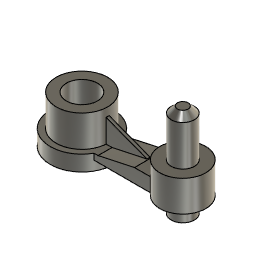
Tarea09_Ej3_jaalobuela (Autodesk Fusion 360 design; units mm, degrees)
Autodesk Fusion 360 part; units mm, degrees
sketch "Sketch1" plane through (0, 0, 0) normal (0, 0, 1) x (1, 0, 0)
  circle A0 centre (-15, 20) radius 8.295
  circle A1 centre (-15, 20) radius 10.195
  line L0 (-15, 20) -> (20.52, 20)
  circle A2 centre (20.52, 20) radius 3.745
  dimension "d1" = 16.59
  dimension "d2" = 20.39
  dimension "d3" = 35.52
  dimension "d4" = 7.49
  constraint concentric A0 A1
  constraint coincident A0.centre A1.centre
  constraint horizontal L0
  constraint coincident L0.end A2.centre
  measures "d1" diameter of A0
  measures "d2" diameter of A1
  measures "d3" distance of A0.centre L0.end
  measures "d4" diameter of A2
extrude "Extrude1" add sketch "Sketch1" along normal blind 5 contours A0 | A1 makes body 1
sketch "Sketch2" plane through (0, 0, 5) normal (0, 0, 1) x (-1, 0, 0)
  circle A0 centre (15, -20) radius 10.195
  circle A1 centre (15, -20) radius 8.295
  dimension "d8" = 16.59
  constraint concentric A0 A1
  measures "d8" diameter of A1
extrude "Extrude2" add sketch "Sketch1" along normal blind 5 separate body contours A2 makes body 2
sketch "Sketch3" plane through (0, 0, 0) normal (0, 0, 1) x (1, 0, 0)
sketch "Sketch4" plane through (0, 0, 0) normal (0, 0, 1) x (1, 0, 0)
sketch "Sketch5" plane through (0, 0, 5) normal (0, 0, 1) x (1, 0, 0)
  circle A0 centre (-15, 20) radius 5
  dimension "d13" = 10
  measures "d13" diameter of A0
sketch "Sketch6" plane through (0, 0, 0) normal (0, 1, 0) x (1, 0, 0)
  circle A0 through (28.49, -40, 0) (25.8725, -40, -1.5112) (25.8725, -40, 1.5112)
  circle A1 through (30.49, -38.0003, 0) (24.8725, -38.0003, -3.2433) (24.8725, -38.0003, 3.2433)
  line L0 (26.745, -40) -> (26.745, -38.0003)
loft "Loft1" add profiles "Sketch6", "Sketch6" section 1 contours A0 in plane through (0, 0, 40) normal (0, 0, -1) section 2 contours A1 in plane through (0, 0, 38.0003) normal (0, 0, -1) separate body makes body 3
extrude "Extrude3" add sketch "Sketch6" along normal blind 13 contours A1 in plane through (0, 0, 38.0003) normal (0, 0, -1) bodies 3
sketch "Sketch7" plane through (0, 0, 0) normal (0, 0, 1) x (1, 0, 0)
  circle A0 centre (48, 1) radius 7.385
  dimension "d21" = 14.77
  measures "d21" diameter of A0
extrude "Extrude4" add sketch "Sketch7" along normal blind 10 separate body makes body 4
move_body "Move1" bodies 4 to x (1, 0, 0) y (0, 1, 0) z (0, 0, 1) at (-21.255, -1, 15.0003)
move_body "Move2" bodies 2 to x (1, 0, 0) y (0, 1, 0) z (0, 0, 1) at (6.225, -20, 10.0003)
move_body "Move3" bodies 2 3 4 to x (1, 0, 0) y (0, 1, 0) z (0, 0, 1) at (-6.225, 20, -10.0003)
sketch "Sketch8" plane through (0, 0, 0) normal (0, 0, 1) x (1, 0, 0)
  line L0 (4, 38) -> (14.58, 38)
  line L1 (14.58, 38) -> (14.58, 28)
  line L2 (14.58, 28) -> (4, 28)
  line L3 (4, 28) -> (4, 38)
  line L4 (15.0651, 15) -> (9.92, 15)
  line L5 (9.92, 15) -> (9.92, 25)
  line L6 (9.92, 25) -> (15.0651, 25)
  circle A0 centre (20.5, 20) radius 7.385
  dimension "d24" = 10.58
  dimension "d25" = 10
  dimension "d28" = 10
  dimension "d31" = 14.77
  dimension "d46" = 10.58
  constraint horizontal L0
  constraint vertical L1
  constraint horizontal L2
  constraint vertical L3
  constraint perpendicular L4 L5
  constraint perpendicular L5 L6
  constraint coincident A0 L6.end
  constraint coincident A0 L4.start
  measures "d24" distance of L0.start L0.end
  measures "d25" distance of L0.start L2.end
  measures "d28" distance of L4.end L5.end
  measures "d31" diameter of A0
  measures "d46" distance of L5 A0.centre
sketch "Sketch9" plane through (0, 0, 0) normal (0, 1, 0) x (1, 0, 0)
  line L0 (13, -5) -> (12.3205, -5)
  line L1 (12.3205, -5) -> (12.3205, -5.53)
  dimension "d30" = 0.53
  constraint horizontal L0
  constraint perpendicular L0 L1
  measures "d30" distance of L0.end L1.end
extrude "Extrude5" add sketch "Sketch8" along normal blind 4.47 separate body contours L4 L5 L6 A0 makes body 5
move_body "Move4" bodies 5 to x (1, 0, 0) y (0, 1, 0) z (0, 0, 1) at (0, 0, 5.53)
sketch "Sketch10" plane through (0, 0, 5) normal (0, 0, 1) x (-1, 0, 0)
  circle A0 centre (15, -20) radius 10.195
  circle A1 centre (15, -20) radius 5
  dimension "d37" = 10
  constraint concentric A0 A1
  measures "d37" diameter of A1
extrude "Extrude6" add sketch "Sketch10" along normal blind 10 contours A1 bodies 1
sketch "Sketch11" plane through (0, 0, 0) normal (0, 1, 0) x (1, 0, 0)
  line L0 (9.92, -5.53) -> (-1.83, -5.53)
  line L1 (9.92, -5.53) -> (9.92, -10)
  line L2 (-1.83, -5.53) -> (-1.83, -7.47)
  line L3 (-1.83, -7.47) -> (9.92, -10)
  dimension "d40" = 11.75
  dimension "d43" = 1.94
  constraint horizontal L0
  constraint perpendicular L0 L1
  constraint perpendicular L0 L2
  measures "d40" distance of L0.start L0.end
  measures "d43" distance of L0.end L2.end
extrude "Extrude7" add sketch "Sketch11" along normal blind 10 separate body makes body 6
move_body "Move5" bodies 6 to x (1, 0, 0) y (0, 1, 0) z (0, 0, 1) at (0, 15, 0)
sketch "Sketch12" plane through (0, 0, 5) normal (0, 0, 1) x (-1, 0, 0)
  circle A0 centre (15, -20) radius 5
  circle A1 centre (15, -20) radius 10.195
  line L0 (15, -20) -> (15, -25)
  line L1 (15, -20) -> (15, -15)
  line L2 (6.1153, -15) -> (1.83, -15)
  line L3 (15, -20) -> (-20.52, -20)
  line L4 (6.1153, -25) -> (1.83, -25)
  arc A2 (6.1153, -15) -> (6.1153, -25) centre (15, -20) ccw
  line L5 (1.83, -15) -> (1.83, -25)
  dimension "d47" = 5
  dimension "d48" = 5
  constraint concentric A0 A2
  constraint coincident A0.centre A1.centre
  constraint vertical L0
  constraint parallel L0 L1
  constraint tangent A0 L2
  constraint perpendicular L1 L2
  constraint symmetric L2.end L3 L4.end
  constraint coincident A1 L4.start
  constraint perpendicular L4 L5
  measures "d47" distance of A0.centre L0.end
  measures "d48" distance of A0.centre L1.end
extrude "Extrude8" add sketch "Sketch12" along normal blind 1.94 separate body contours A1 L2 L3 A2 L5 | A1 L3 L4 A2 L5 makes body 7
move_body "Move6" bodies 7 to x (1, 0, 0) y (0, 1, 0) z (0, 0, 1) at (0, 0, 0.53)
move_body "Move7" bodies 1 to x (1, 0, 0) y (0, 1, 0) z (0, 0, 1) at (0, 0, 2.47)
extrude "Extrude9" add sketch "Sketch1" along normal blind 10 separate body contours A0 makes body 8
move_body "Move8" bodies 8 to x (1, 0, 0) y (0, 1, 0) z (0, 0, 1) at (0, 0, 7.47)
combine "Combine1" operation cut target body 8 tool bodies 1
extrude "Extrude10" add sketch "Sketch1" along normal blind 5 separate body contours A0 | A1 makes body 9
move_body "Move9" bodies 9 to x (1, 0, 0) y (0, 1, 0) z (0, 0, 1) at (0, 0, 2.47)
sketch "Sketch13" plane through (0, 0, 0) normal (0, 1, 0) x (1, 0, 0)
  line L0 (20.52, 0) -> (20.52, 1.5)
  line L1 (20.52, 1.5) -> (9.46, 1.5)
  line L2 (9.46, 1.5) -> (9.46, -12.5848)
  line L3 (-25.195, -2.47) -> (-25.195, -14.93)
  line L4 (-25.195, -14.93) -> (-6.7, -14.93)
  line L5 (-6.7, -14.93) -> (-6.7, -7.47)
  line L6 (-6.7, -7.47) -> (-1.83, -7.47)
  line L7 (-1.83, -7.47) -> (9.46, -9.901)
  line L8 (-6.7, -14.93) -> (9.46, -9.901)
  dimension "d55" = 11.06
  dimension "d56" = 12.46
  dimension "d57" = 7.46
  constraint vertical L0
  constraint perpendicular L0 L1
  constraint perpendicular L1 L2
  constraint vertical L3
  constraint perpendicular L3 L4
  constraint perpendicular L4 L5
  constraint perpendicular L5 L6
  constraint coincident L2 L7.end
  measures "d55" distance of L0.end L1.end
  measures "d56" distance of L3.start L3.end
  measures "d57" distance of L4.end L5.end
extrude "Extrude11" add sketch "Sketch13" along normal blind 1 separate body makes body 10
move_body "Move10" bodies 10 to x (1, 0, 0) y (0, 1, 0) z (0, 0, 1) at (0, 19.5, 0)
copy_body "CopyPasteBodies1" bodies 8 10 3 9 4 2 5 7 6 makes body 11 makes body 12 makes body 13 makes body 14 makes body 15 makes body 16 makes body 17 makes body 18 makes body 19
move_body "Move11" bodies 11 12 13 14 15 16 17 18 19 to x (1, 0, 0) y (0, 1, 0) z (0, 0, 1) at (74, 0, 0)
move_body "Move12" bodies 11 14 to x (1, 0, 0) y (0, 1, 0) z (0, 0, 1) at (2.98, 0, 0)
move_body "Move13" bodies 3 to x (1, 0, 0) y (0, 1, 0) z (0, 0, 1) at (0, 0, 9)
move_body "Move14" bodies 3 to x (1, 0, 0) y (0, 1, 0) z (0, 0, 1) at (0, 0, -9)
combine "Combine2" operation add target body 19 tool bodies 11 18 14 17 12
move_body "Move15" bodies 4 2 3 to x (1, 0, 0) y (0, 1, 0) z (0, 0, 1) at (123, 0, 0)
copy_body "CopyPasteBodies2" bodies 19 makes body 20
move_body "Move16" bodies 20 to x (1, 0, 0) y (0, 1, 0) z (0, 0, 1) at (43, 0, 0)
move_body "Move17" bodies 20 to x (1, 0, 0) y (0, 1, 0) z (0, 0, 1) at (6.02, 0, -0.53)
move_body "Move18" bodies 20 to x (1, 0, 0) y (0, 1, 0) z (0, 0, 1) at (0, 0, 0.53)
move_body "Move19" bodies 20 4 3 2 to x (1, 0, 0) y (0, 1, 0) z (0, 0, 1) at (15, 0, 0)
combine "Combine3" operation add target body 20 tool bodies 4 3 2
copy_body "CopyPasteBodies3" bodies 13 19 16 15 makes body 21 makes body 22 makes body 23 makes body 24
move_body "Move20" bodies 21 22 23 24 to x (1, 0, 0) y (0, 1, 0) z (0, 0, 1) at (150, 0, 0)
sketch "Sketch14" plane through (0, 0, 0) normal (0, 1, 0) x (1, 0, 0)
  line L0 (211, -46) -> (211, -38.54)
  line L1 (211, -46) -> (230.5358, -38.54)
  line L2 (211, -38.54) -> (230.5358, -38.54)
  dimension "d78" = 7.46
  dimension "d79" = 69.1
  constraint vertical L0
  constraint perpendicular L0 L2
  measures "d78" distance of L0.start L0.end
  measures "d79" angle of L0 L1
extrude "Extrude12" add sketch "Sketch14" along normal blind 1 separate body makes body 25
delete_face "DeleteFace1" 1 faces at (225.2966, 19.5, 10.46) on bodies 22
move_body "Move21" bodies 25 to x (1, 0, 0) y (0, 1, 0) z (0, 0, 1) at (11.17, 19.5, -31.07)
move_body "Move22" bodies 25 to x (1, 0, 0) y (0, 1, 0) z (0, 0, 1) at (-1.9, 0, 0)
move_body "Move23" bodies 25 to x (1, 0, 0) y (0, 1, 0) z (0, 0, 1) at (0, 0, 12)
sketch "Sketch15" plane through (0, 0, 0) normal (0, 1, 0) x (1, 0, 0)
  line L0 (240.2606, -16.5373) -> (234.3381, -16.5373)
  line L1 (234.3381, -16.5373) -> (234.3381, -23.6442)
  line L2 (234.3381, -23.6442) -> (240.2606, -23.6442)
  line L3 (240.2606, -23.6442) -> (240.2606, -16.5373)
  constraint horizontal L0
  constraint vertical L1
  constraint horizontal L2
  constraint vertical L3
extrude "Extrude13" cut sketch "Sketch15" along normal blind 33 bodies 25
move_body "Move24" bodies 25 to x (1, 0, 0) y (0, 1, 0) z (0, 0, 1) at (0, 0, -12)
combine "Combine4" operation add target body 23 tool bodies 22 24 25 21 makes body 26 at (220.0919, 21.7331, 14.1367)
combine "Combine5" operation add target body 26 tool bodies 23 makes body 27 at (239.6334, 14.4629, 11.6667)
move_body "Move25" bodies 26 to x (1, 0, 0) y (0, 1, 0) z (0, 0, 1) at (-5, 0, 0)
move_body "Move26" bodies 26 to x (1, 0, 0) y (0, 1, 0) z (0, 0, 1) at (5.02, 0, -0.53)
move_body "Move27" bodies 26 to x (1, 0, 0) y (0, 1, 0) z (0, 0, 1) at (0, 0, 0.53)
combine "Combine6" operation add target body 27 tool bodies 26
move_face "OffsetFaces1" offset 0.13 1 faces at (219.1658, 20.4121, 17.47) on bodies 27
hidden bodies 5 6 7 8 9 10 13 15 16 19 20
